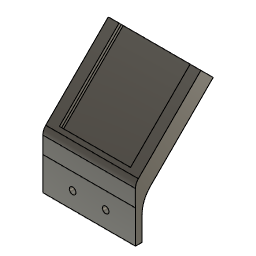
WyzeCamSideRailMount (Autodesk Fusion 360 design; units mm, degrees)
Autodesk Fusion 360 part; units mm, degrees
mesh "Mesh1" [no effect]
sketch "Sketch1" plane through (0, 0, 0) normal (0, 1, 0) x (1, 0, 0)
  line L0 (-2, -27) -> (-52, -27)
  line L1 (-52, -27) -> (-52, -33.6)
  line L2 (-2, -33.4) -> (-2, -27)
  line L3 (1, -25) -> (-55, -25)
  line L4 (-55, -25) -> (-55, -35.5)
  line L5 (1, -35.5) -> (1, -25)
  line L6 (-2, -33.4) -> (-5.5, -33.4)
  line L7 (-5.5, -33.4) -> (-5.5, -35.5)
  line L8 (-5.5, -35.5) -> (1, -35.5)
  line L9 (-52, -33.6) -> (-48.5, -33.6)
  line L10 (-48.5, -33.6) -> (-48.5, -35.5)
  line L11 (-48.5, -35.5) -> (-55, -35.5)
  line L12 (0, 0) -> (-20, 0)
  line L13 (-20, 0) -> (-20, 40)
  line L14 (-20, 40) -> (0, 40)
  line L15 (0, 40) -> (0, 0)
  circle A0 centre (-10, 10) radius 2.1
  circle A1 centre (-10, 30) radius 2.1
  dimension "d1" = 50
  dimension "d2" = 6.4
  dimension "d3" = 4.2
  dimension "d4" = 4.2
  constraint horizontal L0
  constraint vertical L1
  constraint vertical L2
  constraint horizontal L3
  constraint vertical L4
  constraint vertical L5
  constraint perpendicular L2 L6
  constraint perpendicular L6 L7
  constraint perpendicular L5 L8
  constraint perpendicular L1 L9
  constraint perpendicular L9 L10
  constraint perpendicular L4 L11
  constraint horizontal L12
  constraint vertical L13
  constraint horizontal L14
  constraint vertical L15
  constraint coincident L12.start L15.end
  measures "d1" distance of L0.start L0.end
  measures "d2" distance of L0.start L2.start
  measures "d3" diameter of A0
  measures "d4" diameter of A1
extrude "Extrude1" add sketch "Sketch1" along normal blind 51 contours L0 L1 L2 L3 L4 L5 L6 L7 L8 L9 L10 L11 makes body 1
move_body "Move1" bodies 1 to x (1, 0, 0) y (0, 0, 1) z (0, -1, 0) at (0, 25, 25)
move_body "Move2" bodies 1 to x (1, 0, 0) y (0, 1, 0) z (0, 0, 1) at (17, 0, -15)
move_body "Move3" bodies 1 to x (1, 0, 0) y (0, 1, 0) z (0, 0, 1) at (0, 7, 0)
sketch "Sketch7" plane through (0, 0, 0) normal (0, 1, 0) x (1, 0, 0)
  spline S0 degree 5 poles (-4, 0) (-3.9494, -0.2229) (-3.9201, -0.6464) (-4.1375, -1.1978) (-5.088, -1.7004) (-7.2158, -1.9004) (-9.9029, -1.6818) (-12.6226, -1.104) (-14.8672, -0.2446) (-16.2644, 0.8173) (-16.7411, 2.0267) (-16.4614, 3.3493) (-15.7161, 4.7618) (-14.8322, 6.2444) (-14.0677, 7.7724) (-13.5324, 9.3094) (-13.2287, 10.8105) (-13.0766, 12.2246) (-12.945, 13.4967) (-12.6795, 14.5705) (-12.1312, 15.3901) (-11.1911, 15.9081) (-9.8236, 16.0926) (-8.1057, 15.9368) (-6.249, 15.4637) (-4.5268, 14.7174) (-3.2157, 13.7547) (-2.5287, 12.6368) (-2.558, 11.4219) (-3.1969, 10.156) (-4.1935, 8.8717) (-5.2314, 7.5895) (-6.0053, 6.3177) (-6.2904, 5.0529) (-6.0329, 3.7792) (-5.3402, 2.4827) (-4.6537, 1.4443) (-4.2238, 0.6912) (-4.0506, 0.2229) (-4, 0) knots 0 0 0 0 0 0 0.028571 0.057143 0.085714 0.114286 0.142857 0.171429 0.2 0.228571 0.257143 0.285714 0.314286 0.342857 0.371429 0.4 0.428571 0.457143 0.485714 0.514286 0.542857 0.571429 0.6 0.628571 0.657143 0.685714 0.714286 0.742857 0.771429 0.8 0.828571 0.857143 0.885714 0.914286 0.942857 0.971429 1 1 1 1 1 1
  line L0 (0, 0) -> (0, 15)
  spline S1 degree 5 poles (4, 0) (3.9494, -0.2229) (3.9201, -0.6464) (4.1375, -1.1978) (5.088, -1.7004) (7.2158, -1.9004) (9.9029, -1.6818) (12.6226, -1.104) (14.8672, -0.2446) (16.2644, 0.8173) (16.7411, 2.0267) (16.4614, 3.3493) (15.7161, 4.7618) (14.8322, 6.2444) (14.0677, 7.7724) (13.5324, 9.3094) (13.2287, 10.8105) (13.0766, 12.2246) (12.945, 13.4967) (12.6795, 14.5705) (12.1312, 15.3901) (11.1911, 15.9081) (9.8236, 16.0926) (8.1057, 15.9368) (6.249, 15.4637) (4.5268, 14.7174) (3.2157, 13.7547) (2.5287, 12.6368) (2.558, 11.4219) (3.1969, 10.156) (4.1935, 8.8717) (5.2314, 7.5895) (6.0053, 6.3177) (6.2904, 5.0529) (6.0329, 3.7792) (5.3402, 2.4827) (4.6537, 1.4443) (4.2238, 0.6912) (4.0506, 0.2229) (4, 0) knots 0 0 0 0 0 0 0.028571 0.057143 0.085714 0.114286 0.142857 0.171429 0.2 0.228571 0.257143 0.285714 0.314286 0.342857 0.371429 0.4 0.428571 0.457143 0.485714 0.514286 0.542857 0.571429 0.6 0.628571 0.657143 0.685714 0.714286 0.742857 0.771429 0.8 0.828571 0.857143 0.885714 0.914286 0.942857 0.971429 1 1 1 1 1 1
  line L1 (-4.2874, 1.266) -> (-3.7126, -1.266)
  line L2 (4.2874, 1.266) -> (3.7126, -1.266)
  point P0 (-15, 0)
  point P1 (-15, 6)
  point P2 (-12.8913, 13.5549)
  point P3 (-10, 16)
  point P4 (-2.6541, 12.3795)
  point P5 (-6, 6)
  point P6 (15, 6)
  point P7 (2.6541, 12.3795)
  point P8 (15, 0)
  point P9 (10, 16)
  point P10 (6, 6)
  point P11 (12.8913, 13.5549)
  constraint coincident L0.start origin
  constraint vertical L0
  constraint midpoint S0.start L1
  constraint symmetric S0.start L0 S1.start
  constraint symmetric P0 L0 P8
  constraint symmetric P1 L0 P6
  constraint symmetric P2 L0 P11
  constraint symmetric P3 L0 P9
  constraint symmetric P4 L0 P7
  constraint symmetric P5 L0 P10
  constraint symmetric L0 L1.start L2.start
  constraint symmetric L0 L1.end L2.end
move_body "Move9" bodies 1 to x (1, 0, 0) y (0, 1, 0) z (0, 0, 1) at (10, 0, 0)
box "BoxPrimitive2" add length 10.5 width 56 height 5 placed x (0, 1, 0) y (1, 0, 0) z (0, 0, -1) at (-28, -3.5, -40) separate body makes body 2
move_body "Move12" bodies 2 to x (1, 0, 0) y (0, 1, 0) z (0, 0, 1) at (0, 0, 50)
move_body "Move14" bodies 2 1 to x (1, 0, 0) y (0, 0.707107, -0.707107) z (0, 0.707107, 0.707107) at (0, -21.0751, 11.6705)
move_body "Move15" bodies 2 1 to x (1, 0, 0) y (0, 1, 0) z (0, 0, 1) at (0, 20, 0)
move_body "Move16" bodies 1 2 to x (1, 0, 0) y (0, 1, 0) z (0, 0, 1) at (0, 0, -25)
sketch "Sketch10" plane through (0, 0, 0) normal (0, 1, 0) x (1, 0, 0)
  line L0 (-28, 20) -> (28, 20)
  line L1 (28, 20) -> (28, 40)
  line L2 (28, 40) -> (-28, 40)
  line L3 (-28, 40) -> (-28, 20)
  circle A0 centre (-10, 30) radius 2
  circle A1 centre (10, 30) radius 2
  constraint horizontal L0
  constraint vertical L1
  constraint horizontal L2
  constraint vertical L3
extrude "Extrude4" add sketch "Sketch10" along normal blind 4 separate body makes body 3
loft "Loft4" add section 1 face at (9.3333, 4.9353, -12.2688) section 2 face at (-9.3333, 1.3333, -20) on bodies 2 3 bodies 2 3
combine "Combine4" operation add target body 1 tool bodies 2
fillet "Fillet5" radius 6 1 edges at (0, -0.0144, -7.3191) on bodies 1
fillet "Fillet6" radius 17.5 2 edges at (0, 7.4102, -14.7437) (0, 4, -20) on bodies 1
